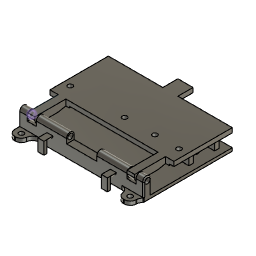
assembly (Autodesk Fusion 360 archive; units mm, degrees)
design "bottom"
Autodesk Fusion 360 part; units mm, degrees
(part 1 of 2)
sketch "Sketch1" plane through (0, 0, 0) normal (0, 0, 1) x (1, 0, 0)
  line L0 (325.5222, -11.5288) -> (325.5222, -23.0288)
  line L1 (309.5222, -20.1288) -> (309.5222, -14.4288)
  line L2 (192.5197, -2.0788) -> (192.5197, -69.9533) construction
  line L3 (325.5222, -11.5288) -> (316.5222, -11.5288)
  line L4 (325.5222, -23.0288) -> (316.5222, -23.0288)
  line L5 (334.5222, -14.4288) -> (343.2222, -14.4288)
  line L6 (350.5222, -11.5288) -> (350.5222, -23.0288)
  line L7 (334.5222, -20.1288) -> (334.5222, -14.4288)
  line L8 (343.2222, -20.1288) -> (343.2222, -23.0288)
  line L9 (350.5222, -11.5288) -> (343.2222, -11.5288)
  line L10 (343.2222, -14.4288) -> (343.2222, -11.5288)
  line L11 (334.5222, -20.1288) -> (343.2222, -20.1288)
  line L12 (350.5222, -23.0288) -> (343.2222, -23.0288)
  line L13 (367.5222, -87.072) -> (367.5222, -157.1728)
  line L14 (327.5222, -47.072) -> (317.8871, -47.072)
  line L15 (312.8871, -42.072) -> (312.8871, -37.072)
  line L16 (317.8871, -32.072) -> (372.5422, -32.072)
  arc A0 (317.8871, -32.072) -> (312.8871, -37.072) centre (317.8871, -37.072) ccw
  arc A1 (312.8871, -42.072) -> (317.8871, -47.072) centre (317.8871, -42.072) ccw
  arc A2 (367.5222, -87.072) -> (327.5222, -47.072) centre (327.5222, -87.072) ccw
  arc A3 (284.5222, -240.1728) -> (367.5222, -157.1728) centre (284.5222, -157.1728) ccw
  line L17 (67.1522, -32.072) -> (12.4972, -32.072)
  arc A4 (72.1522, -37.072) -> (67.1522, -32.072) centre (67.1522, -37.072) ccw
  line L18 (72.1522, -42.072) -> (72.1522, -37.072)
  arc A5 (67.1522, -47.072) -> (72.1522, -42.072) centre (67.1522, -42.072) ccw
  line L19 (57.5171, -47.072) -> (67.1522, -47.072)
  arc A6 (57.5171, -47.072) -> (17.5171, -87.072) centre (57.5171, -87.072) ccw
  line L20 (17.5171, -87.072) -> (17.5171, -157.1728)
  arc A7 (17.5171, -157.1728) -> (100.5171, -240.1728) centre (100.5171, -157.1728) ccw
  line L21 (316.5222, -11.5288) -> (314.4916, -14.4288)
  line L22 (316.5222, -11.5288) -> (320.409, -11.5288) construction
  line L23 (309.5222, -20.1288) -> (314.4916, -20.1288)
  line L24 (314.4916, -20.1288) -> (316.5222, -23.0288)
  line L25 (314.4916, -14.4288) -> (309.5222, -14.4288)
  circle A8 centre (362.5222, -10.5788) radius 3
  circle A9 centre (362.5222, -23.572) radius 3
  circle A10 centre (373.5222, -17.0788) radius 4
  line L26 (360.5472, -12.837) -> (360.5472, -21.3138)
  circle A11 centre (278.8372, -196.4356) radius 3
  circle A12 centre (278.8372, -209.4287) radius 3
  circle A13 centre (267.8372, -202.9356) radius 4
  line L27 (280.8122, -198.6937) -> (280.8122, -207.1706)
  circle A14 centre (253.8372, -209.4287) radius 3
  circle A15 centre (253.8372, -196.4356) radius 3
  circle A16 centre (242.8372, -202.9356) radius 4
  line L28 (255.8122, -198.6937) -> (255.8122, -207.1706)
  circle A17 centre (303.8372, -209.4287) radius 3
  circle A18 centre (303.8372, -196.4356) radius 3
  circle A19 centre (292.8372, -202.9356) radius 4
  line L29 (305.8122, -198.6937) -> (305.8122, -207.1706)
  line L30 (372.5422, -32.072) -> (372.5222, -32.072)
  line L31 (382.5222, -22.072) -> (382.5222, -12.0576)
  line L32 (372.5222, -2.0576) -> (372.5422, -2.0576)
  arc A20 (382.5222, -12.0576) -> (372.5222, -2.0576) centre (372.5222, -12.0576) ccw
  arc A21 (372.5222, -32.072) -> (382.5222, -22.072) centre (372.5222, -22.072) ccw
  arc A22 (12.5171, -2.0576) -> (2.5171, -12.0576) centre (12.5171, -12.0576) ccw
  line L33 (2.5171, -22.072) -> (2.5171, -12.0576)
  arc A23 (2.5171, -22.072) -> (12.5171, -32.072) centre (12.5171, -22.072) ccw
  line L34 (284.5222, -240.1728) -> (100.5171, -240.1728)
  line L35 (12.5171, -2.0576) -> (372.5422, -2.0576)
  line L36 (133.9354, -11.0576) -> (139.9354, -11.0576)
  line L37 (142.3054, -15.8969) -> (141.8063, -16.54)
  line L38 (144.1763, -21.3793) -> (157.1763, -21.3793)
  line L39 (159.6876, -16.7381) -> (159.0084, -15.6988)
  line L40 (161.5197, -11.0576) -> (167.5197, -11.0576)
  arc A24 (142.3054, -15.8969) -> (139.9354, -11.0576) centre (139.9354, -14.0576) ccw
  arc A25 (161.5197, -11.0576) -> (159.0084, -15.6988) centre (161.5197, -14.0576) ccw
  arc A26 (157.1763, -21.3793) -> (159.6876, -16.7381) centre (157.1763, -18.3793) ccw
  arc A27 (141.8063, -16.54) -> (144.1763, -21.3793) centre (144.1763, -18.3793) ccw
  arc A28 (226.0309, -15.6988) -> (223.5197, -11.0576) centre (223.5197, -14.0576) ccw
  arc A29 (240.863, -21.3793) -> (243.233, -16.54) centre (240.863, -18.3793) ccw
  line L41 (240.863, -21.3793) -> (227.863, -21.3793)
  line L42 (242.7339, -15.8969) -> (243.233, -16.54)
  arc A30 (245.1039, -11.0576) -> (242.7339, -15.8969) centre (245.1039, -14.0576) ccw
  line L43 (223.5197, -11.0576) -> (217.5197, -11.0576)
  line L44 (225.3517, -16.7381) -> (226.0309, -15.6988)
  line L45 (251.1039, -11.0576) -> (245.1039, -11.0576)
  arc A31 (225.3517, -16.7381) -> (227.863, -21.3793) centre (227.863, -18.3793) ccw
  line L46 (315.4335, -32.7154) -> (320, -31)
  line L47 (242.8372, -198.9356) -> (242.8372, -206.9356) construction
  line L48 (238.8372, -202.9356) -> (246.8372, -202.9356) construction
  line L49 (250.8372, -196.4356) -> (256.8372, -196.4356) construction
  line L50 (253.8372, -193.4356) -> (253.8372, -199.4356) construction
  line L51 (253.8372, -206.4287) -> (253.8372, -212.4287) construction
  line L52 (250.8372, -209.4287) -> (256.8372, -209.4287) construction
  line L53 (263.8372, -202.9356) -> (271.8372, -202.9356) construction
  line L54 (267.8372, -198.9356) -> (267.8372, -206.9356) construction
  line L55 (275.8372, -196.4356) -> (281.8372, -196.4356) construction
  line L56 (278.8372, -193.4356) -> (278.8372, -199.4356) construction
  line L57 (278.8372, -206.4287) -> (278.8372, -212.4287) construction
  line L58 (275.8372, -209.4287) -> (281.8372, -209.4287) construction
  line L59 (288.8372, -202.9356) -> (296.8372, -202.9356) construction
  line L60 (292.8372, -198.9356) -> (292.8372, -206.9356) construction
  line L61 (300.8372, -196.4356) -> (306.8372, -196.4356) construction
  line L62 (303.8372, -193.4356) -> (303.8372, -199.4356) construction
  line L63 (303.8372, -206.4287) -> (303.8372, -212.4287) construction
  line L64 (300.8372, -209.4287) -> (306.8372, -209.4287) construction
  line L65 (92.2021, -198.9356) -> (92.2021, -206.9356) construction
  line L66 (109.2021, -209.4287) -> (103.2021, -209.4287) construction
  line L67 (142.2021, -198.9356) -> (142.2021, -206.9356) construction
  line L68 (131.2021, -206.4287) -> (131.2021, -212.4287) construction
  line L69 (109.2021, -196.4356) -> (103.2021, -196.4356) construction
  line L70 (131.2021, -193.4356) -> (131.2021, -199.4356) construction
  circle A32 centre (131.2021, -196.4356) radius 3
  circle A33 centre (142.2021, -202.9356) radius 4
  circle A34 centre (117.2021, -202.9356) radius 4
  line L71 (104.2271, -198.6937) -> (104.2271, -207.1706)
  line L72 (81.2021, -193.4356) -> (81.2021, -199.4356) construction
  line L73 (106.2021, -206.4287) -> (106.2021, -212.4287) construction
  line L74 (106.2021, -193.4356) -> (106.2021, -199.4356) construction
  line L75 (96.2021, -202.9356) -> (88.2021, -202.9356) construction
  line L76 (134.2021, -196.4356) -> (128.2021, -196.4356) construction
  line L77 (79.2271, -198.6937) -> (79.2271, -207.1706)
  line L78 (117.2021, -198.9356) -> (117.2021, -206.9356) construction
  circle A35 centre (106.2021, -196.4356) radius 3
  line L79 (81.2021, -206.4287) -> (81.2021, -212.4287) construction
  line L80 (134.2021, -209.4287) -> (128.2021, -209.4287) construction
  circle A36 centre (81.2021, -196.4356) radius 3
  circle A37 centre (92.2021, -202.9356) radius 4
  line L81 (84.2021, -209.4287) -> (78.2021, -209.4287) construction
  circle A38 centre (131.2021, -209.4287) radius 3
  line L82 (84.2021, -196.4356) -> (78.2021, -196.4356) construction
  line L83 (129.2271, -198.6937) -> (129.2271, -207.1706)
  circle A39 centre (106.2021, -209.4287) radius 3
  line L84 (146.2021, -202.9356) -> (138.2021, -202.9356) construction
  circle A40 centre (81.2021, -209.4287) radius 3
  line L85 (121.2021, -202.9356) -> (113.2021, -202.9356) construction
  line L86 (362.5222, -20.572) -> (362.5222, -26.572) construction
  line L87 (359.5222, -23.572) -> (365.5222, -23.572) construction
  line L88 (373.5221, -13.0788) -> (373.5221, -21.0788) construction
  line L89 (369.5222, -17.0788) -> (377.5222, -17.0788) construction
  line L90 (362.5222, -7.5788) -> (362.5222, -13.5788) construction
  line L91 (359.5222, -10.5788) -> (365.5222, -10.5788) construction
  line L92 (59.5171, -23.0288) -> (68.5171, -23.0288)
  line L93 (22.5171, -20.572) -> (22.5171, -26.572) construction
  line L94 (11.5172, -13.0788) -> (11.5172, -21.0788) construction
  line L95 (34.5171, -11.5288) -> (41.8171, -11.5288)
  line L96 (25.5171, -10.5788) -> (19.5171, -10.5788) construction
  line L97 (34.5171, -23.0288) -> (41.8171, -23.0288)
  line L98 (59.5171, -11.5288) -> (68.5171, -11.5288)
  line L99 (34.5171, -11.5288) -> (34.5171, -23.0288)
  circle A41 centre (22.5171, -23.572) radius 3
  circle A42 centre (11.5171, -17.0788) radius 4
  line L100 (75.5171, -20.1288) -> (75.5171, -14.4288)
  line L101 (25.5171, -23.572) -> (19.5171, -23.572) construction
  line L102 (50.5171, -14.4288) -> (41.8171, -14.4288)
  line L103 (68.5171, -11.5288) -> (64.6303, -11.5288) construction
  line L104 (70.5477, -14.4288) -> (75.5171, -14.4288)
  line L105 (70.5477, -20.1288) -> (68.5171, -23.0288)
  line L106 (22.5171, -7.5788) -> (22.5171, -13.5788) construction
  line L107 (75.5171, -20.1288) -> (70.5477, -20.1288)
  line L108 (41.8171, -20.1288) -> (41.8171, -23.0288)
  line L109 (68.5171, -11.5288) -> (70.5477, -14.4288)
  line L110 (24.4921, -12.837) -> (24.4921, -21.3138)
  line L111 (15.5171, -17.0788) -> (7.5171, -17.0788) construction
  line L112 (50.5171, -20.1288) -> (41.8171, -20.1288)
  line L113 (50.5171, -20.1288) -> (50.5171, -14.4288)
  line L114 (59.5171, -11.5288) -> (59.5171, -23.0288)
  circle A43 centre (22.5171, -10.5788) radius 3
  line L115 (41.8171, -14.4288) -> (41.8171, -11.5288)
  point P0 (309.5222, -17.2788)
  point P1 (325.5222, -17.2788)
  point P2 (325.5222, -17.2788)
  point P3 (309.5222, -17.2788)
  point P4 (350.5222, -17.2788)
  point P5 (334.5222, -17.2788)
  point P6 (350.5222, -17.2788)
  point P7 (334.5222, -17.2788)
  point P8 (330.5222, -17.0788)
  point P9 (314.5222, -17.0788)
  point P10 (330.5222, -17.0788)
  point P11 (314.5222, -17.0788)
  point P12 (359.5472, -10.1923)
  point P13 (359.5433, -23.9267)
  point P14 (281.8162, -209.7835)
  point P15 (281.8122, -196.0491)
  point P16 (256.8122, -196.0491)
  point P17 (256.8162, -209.7835)
  point P18 (306.8122, -196.0491)
  point P19 (306.8162, -209.7835)
  point P20 (192.5197, -240.1728)
  point P21 (128.2231, -209.7835)
  point P22 (78.2271, -196.0491)
  point P23 (103.2271, -196.0491)
  point P24 (103.2231, -209.7835)
  point P25 (128.2271, -196.0491)
  point P26 (78.2231, -209.7835)
  point P27 (59.5171, -17.2788)
  point P28 (54.5171, -17.0788)
  point P29 (12.5171, -22.072)
  point P30 (59.5171, -17.2788)
  point P31 (34.5171, -17.2788)
  point P32 (50.5171, -17.2788)
  point P33 (70.5171, -17.0788)
  point P34 (70.5171, -17.0788)
  point P35 (34.5171, -17.2788)
  point P36 (50.5171, -17.2788)
  point P37 (12.5171, -12.0576)
  point P38 (25.4921, -10.1923)
  point P39 (25.496, -23.9267)
  point P40 (75.5171, -17.2788)
  point P41 (75.5171, -17.2788)
  point P42 (54.5171, -17.0788)
  dimension "d16" = 5.7
  dimension "d20" = 11.5
  dimension "d25" = 16
  dimension "d27" = 9
  dimension "d28" = 9
  dimension "d33" = 5.7
  dimension "d34" = 11.5
  dimension "d35" = 16
  dimension "d36" = 7.3
  dimension "d37" = 7.3
  dimension "d39" = 25
  dimension "d48" = 5
  dimension "d49" = 5
  dimension "d50" = 40
  dimension "d57" = 15
  dimension "d67" = 125
  dimension "d68" = 125
  dimension "d80" = 6
  dimension "d81" = 6
  dimension "d83" = 8.5
  dimension "d85" = 8
  dimension "d95" = 1
  dimension "d98" = 25
  dimension "d99" = 0
  dimension "d101" = 10
  dimension "d102" = 10
  dimension "d122" = 32
  dimension "d123" = 3
  dimension "d124" = 3
  dimension "d125" = 3
  dimension "d126" = 3
  dimension "d127" = 9
  dimension "d128" = 9
  dimension "d129" = 6
  dimension "d130" = 6
  dimension "d131" = 13
  constraint vertical L0
  constraint vertical L1
  constraint midpoint L1 P3
  constraint midpoint L0 P2
  constraint coincident P2 P1
  constraint coincident P3 P0
  constraint horizontal P2 P3
  constraint perpendicular L0 L3
  constraint perpendicular L0 L4
  constraint vertical L6
  constraint vertical L7
  constraint midpoint P7 L7
  constraint midpoint P6 L6
  constraint coincident P6 P4
  constraint coincident P7 P5
  constraint horizontal P6 P7
  constraint perpendicular L6 L9
  constraint perpendicular L6 L12
  constraint perpendicular L7 L11
  constraint perpendicular L8 L12
  constraint perpendicular L5 L7
  constraint perpendicular L9 L10
  constraint coincident P10 P8
  constraint coincident P11 P9
  constraint horizontal P10 P11
  constraint perpendicular L15 L16
  constraint perpendicular L14 L15
  constraint tangent L15 A0
  constraint tangent L16 A0
  constraint tangent L15 A1
  constraint tangent L14 A1
  constraint tangent L13 A2
  constraint tangent L14 A2
  constraint horizontal L16
  constraint tangent L13 A3
  constraint symmetric L16.end L2 L17.end
  constraint symmetric L2 L15.end A4.start
  constraint symmetric L2 L16.start L17.start
  constraint symmetric L2 A0 A4
  constraint symmetric L2 L15.start L18.start
  constraint symmetric L2 L14.end A5.start
  constraint symmetric L2 A1 A5
  constraint symmetric L2 L13.start A6.end
  constraint symmetric L2 L14.start L19.start
  constraint symmetric L2 A2 A6
  constraint symmetric L2 L13.end L20.end
  constraint symmetric L2 A3.start A7.end
  constraint symmetric L2 A3 A7
  constraint horizontal L22
  constraint perpendicular L1 L23
  constraint perpendicular L1 L25
  constraint vertical A8.centre A9.centre
  constraint coincident A8 P12
  constraint coincident A9 P13
  constraint coincident A8 L26.start
  constraint coincident A9 L26.end
  constraint vertical L26
  constraint perpendicular L31 L32
  constraint tangent L31 A20
  constraint tangent L32 A20
  constraint tangent L30 A21
  constraint tangent L31 A21
  constraint symmetric L2 L31.end A22.end
  constraint symmetric L2 L32.start A22.start
  constraint symmetric L2 A20 A22
  constraint symmetric L2 L30.end A23.end
  constraint symmetric L2 L31.start L33.start
  constraint symmetric L2 A21 A23
  constraint tangent A7 L34
  constraint tangent A20 L35
  constraint midpoint L34 P20
  constraint horizontal L36
  constraint parallel L36 L38
  constraint parallel L38 L40
  constraint tangent L36 A24
  constraint tangent L37 A24
  constraint tangent L40 A25
  constraint tangent L39 A25
  constraint tangent L38 A26
  constraint tangent L39 A26
  constraint tangent L37 A27
  constraint tangent L38 A27
  constraint symmetric L2 L36.start L45.start
  constraint symmetric L2 L40.end L43.end
  constraint symmetric L2 L36.end A30.start
  constraint symmetric L2 L37.start L42.start
  constraint symmetric L2 A24 A30
  constraint symmetric L2 L40.start A28.end
  constraint symmetric L2 L39.end A28.start
  constraint symmetric L2 A25 A28
  constraint symmetric L2 L38.end L41.end
  constraint symmetric L2 L39.start L44.start
  constraint symmetric L2 A26 A31
  constraint symmetric L2 L37.end A29.end
  constraint symmetric L2 L38.start A29.start
  constraint symmetric L2 A27 A29
  constraint coincident A0 L46.start
  constraint coincident A16 L47.start
  constraint coincident A16 L47.end
  constraint vertical L47
  constraint coincident A16 L48.start
  constraint coincident A16 L48.end
  constraint perpendicular L47 L48
  constraint coincident A15 L49.start
  constraint coincident A15 L49.end
  constraint horizontal L49
  constraint coincident A15 L50.start
  constraint coincident A15 L50.end
  constraint perpendicular L49 L50
  constraint coincident A14 L51.start
  constraint coincident A14 L51.end
  constraint parallel L28 L51
  constraint coincident A14 L52.start
  constraint coincident A14 L52.end
  constraint perpendicular L51 L52
  constraint coincident A13 L53.start
  constraint coincident A13 L53.end
  constraint horizontal L53
  constraint coincident A13 L54.start
  constraint coincident A13 L54.end
  constraint perpendicular L53 L54
  constraint coincident A11 L55.start
  constraint coincident A11 L55.end
  constraint horizontal L55
  constraint coincident A11 L56.start
  constraint coincident A11 L56.end
  constraint perpendicular L55 L56
  constraint coincident A12 L57.start
  constraint coincident A12 L57.end
  constraint perpendicular L55 L57
  constraint coincident A12 L58.start
  constraint coincident A12 L58.end
  constraint perpendicular L57 L58
  constraint coincident A19 L59.start
  constraint coincident A19 L59.end
  constraint horizontal L59
  constraint coincident A19 L60.start
  constraint coincident A19 L60.end
  constraint perpendicular L59 L60
  constraint coincident A18 L61.start
  constraint coincident A18 L61.end
  constraint horizontal L61
  constraint coincident A18 L62.start
  constraint coincident A18 L62.end
  constraint perpendicular L61 L62
  constraint coincident A17 L63.start
  constraint coincident A17 L63.end
  constraint perpendicular L61 L63
  constraint coincident A17 L64.start
  constraint coincident A17 L64.end
  constraint perpendicular L63 L64
  constraint symmetric L2 L27.start L71.start
  constraint symmetric L2 L27.end L71.end
  constraint symmetric L2 P14 P24
  constraint symmetric L2 P15 P23
  constraint symmetric L2 A11 A35
  constraint symmetric L2 A12 A39
  constraint symmetric L2 A13 A34
  constraint symmetric L2 L28.end L83.end
  constraint symmetric L2 P16 P25
  constraint symmetric L2 A14 A38
  constraint symmetric L2 L28.start L83.start
  constraint symmetric L2 A15 A32
  constraint symmetric L2 A16 A33
  constraint symmetric L2 P17 P21
  constraint symmetric L2 L29.end L77.end
  constraint symmetric L2 P18 P22
  constraint symmetric L2 A17 A40
  constraint symmetric L2 L29.start L77.start
  constraint symmetric L2 A18 A36
  constraint symmetric L2 A19 A37
  constraint symmetric L2 P19 P26
  constraint symmetric L2 L47.start L67.start
  constraint symmetric L2 L47.end L67.end
  constraint symmetric L2 L48.start L84.start
  constraint symmetric L2 L48.end L84.end
  constraint symmetric L2 L49.start L76.start
  constraint symmetric L2 L49.end L76.end
  constraint symmetric L2 L50.start L70.start
  constraint symmetric L2 L50.end L70.end
  constraint symmetric L2 L51.start L68.start
  constraint symmetric L2 L51.end L68.end
  constraint symmetric L2 L52.start L80.start
  constraint symmetric L2 L52.end L80.end
  constraint symmetric L2 L53.start L85.start
  constraint symmetric L2 L53.end L85.end
  constraint symmetric L2 L54.start L78.start
  constraint symmetric L2 L54.end L78.end
  constraint symmetric L2 L55.start L69.start
  constraint symmetric L2 L55.end L69.end
  constraint symmetric L2 L56.start L74.start
  constraint symmetric L2 L56.end L74.end
  constraint symmetric L2 L57.start L73.start
  constraint symmetric L2 L57.end L73.end
  constraint symmetric L2 L58.start L66.start
  constraint symmetric L2 L58.end L66.end
  constraint symmetric L2 L59.start L75.start
  constraint symmetric L2 L59.end L75.end
  constraint symmetric L2 L60.start L65.start
  constraint symmetric L2 L60.end L65.end
  constraint symmetric L2 L61.start L82.start
  constraint symmetric L2 L61.end L82.end
  constraint symmetric L2 L62.start L72.start
  constraint symmetric L2 L62.end L72.end
  constraint symmetric L2 L63.start L79.start
  constraint symmetric L2 L63.end L79.end
  constraint symmetric L2 L64.start L81.start
  constraint symmetric L2 L64.end L81.end
  constraint coincident A9 L86.start
  constraint coincident A9 L86.end
  constraint vertical L86
  constraint coincident A9 L87.start
  constraint coincident A9 L87.end
  constraint perpendicular L86 L87
  constraint coincident A10 L88.start
  constraint coincident A10 L88.end
  constraint perpendicular L87 L88
  constraint coincident A10 L89.start
  constraint coincident A10 L89.end
  constraint perpendicular L88 L89
  constraint coincident A8 L90.start
  constraint coincident A8 L90.end
  constraint vertical L90
  constraint coincident A8 L91.start
  constraint coincident A8 L91.end
  constraint perpendicular L90 L91
  constraint symmetric L1.end L2 L100.end
  constraint symmetric L0.start L2 L98.start
  constraint symmetric L1.start L2 L100.start
  constraint symmetric L2 L0.end L92.start
  constraint symmetric L2 P3 P41
  constraint symmetric L2 P2 P30
  constraint symmetric L2 L3.end L98.end
  constraint symmetric L2 L4.end L92.end
  constraint symmetric L2 P6 P35
  constraint symmetric L2 L6.start L95.start
  constraint symmetric L2 L5.start L102.start
  constraint symmetric L2 L7.start L112.start
  constraint symmetric L2 L6.end L97.start
  constraint symmetric L2 P7 P36
  constraint symmetric L2 L5.end L102.end
  constraint symmetric L2 L8.start L108.start
  constraint symmetric L2 L8.end L97.end
  constraint symmetric L2 L9.end L95.end
  constraint symmetric L2 P10 P42
  constraint symmetric L2 P11 P34
  constraint symmetric L2 L21.end L104.start
  constraint symmetric L2 L22.end L103.end
  constraint symmetric L2 L23.end L105.start
  constraint symmetric L2 A8 A43
  constraint symmetric L2 A9 A41
  constraint symmetric L2 A10 A42
  constraint symmetric L2 P12 P38
  constraint symmetric L2 P13 P39
  constraint symmetric L2 L26.start L110.start
  constraint symmetric L2 L26.end L110.end
  constraint symmetric L2 A20.centre P37
  constraint symmetric L2 A21.centre P29
  constraint symmetric L2 L86.start L93.start
  constraint symmetric L2 L86.end L93.end
  constraint symmetric L2 L87.start L101.start
  constraint symmetric L2 L87.end L101.end
  constraint symmetric L2 L88.start L94.start
  constraint symmetric L2 L88.end L94.end
  constraint symmetric L2 L89.start L111.start
  constraint symmetric L2 L89.end L111.end
  constraint symmetric L2 L90.start L106.start
  constraint symmetric L2 L90.end L106.end
  constraint symmetric L2 L91.start L96.start
  constraint symmetric L2 L91.end L96.end
  measures "d16" distance of L1.end L1.start
  measures "d20" distance of L0.start L0.end
  measures "d25" distance of L0 L1
  measures "d27" distance of L0.start L3.end
  measures "d28" distance of L0.end L4.end
  measures "d33" distance of L5.start L7.start
  measures "d34" distance of L6.start L6.end
  measures "d35" distance of L6 L7
  measures "d36" distance of L6.start L9.end
  measures "d37" distance of L6.end L8.end
  measures "d39" distance of L0.end L6.end
  measures "d48" radius of A0
  measures "d49" radius of A1
  measures "d50" radius of A2
  measures "d57" distance of L14 L16
  measures "d67" angle of L21 L22
  measures "d68" angle of L4 L24
  measures "d80" diameter of A8
  measures "d81" diameter of A9
  measures "d83" distance of L16 A9.centre
  measures "d85" diameter of A10
  measures "d95" distance of P12 L26
  measures "d101" radius of A20
  measures "d102" radius of A21
  measures "d122" distance of L6 L31
  measures "d123" radius of A24
  measures "d124" radius of A25
  measures "d125" radius of A26
  measures "d126" radius of A27
  measures "d127" distance of L35 L36
  measures "d128" distance of L35 L40
  measures "d129" distance of L36.start L36.end
  measures "d130" distance of L40.end L40.start
  measures "d131" distance of L38.end L38.start
sketch "Sketch2" plane through (0, 0, 0) normal (0, 0, 1) x (1, 0, 0)
  circle A0 centre (81.2021, -196.4356) radius 3
  circle A1 centre (81.2021, -209.4287) radius 3
  circle A2 centre (92.2021, -202.9356) radius 4
  circle A3 centre (106.2021, -196.4356) radius 3
  circle A4 centre (106.2021, -209.4287) radius 3
  circle A5 centre (117.2021, -202.9356) radius 4
  circle A6 centre (131.2021, -196.4356) radius 3
  circle A7 centre (131.2021, -209.4287) radius 3
  circle A8 centre (142.2021, -202.9356) radius 4
  line L0 (79.2271, -198.6937) -> (79.2271, -207.1706)
  line L1 (104.2271, -198.6937) -> (104.2271, -207.1706)
  line L2 (129.2271, -198.6937) -> (129.2271, -207.1706)
  circle A9 centre (81.2021, -196.4356) radius 2.8
  circle A10 centre (81.2021, -209.4287) radius 2.8
  circle A11 centre (92.2021, -202.9356) radius 3.8
  circle A12 centre (106.2021, -196.4356) radius 2.8
  circle A13 centre (106.2021, -209.4287) radius 2.8
  circle A14 centre (117.2021, -202.9356) radius 3.8
  circle A15 centre (131.2021, -209.4287) radius 2.8
  circle A16 centre (131.2021, -196.4356) radius 2.8
  circle A17 centre (142.2021, -202.9356) radius 3.8
  dimension "d152" = -0.2
  dimension "d154" = 0.2
  dimension "d155" = 0.2
  constraint concentric A1 A10
  constraint concentric A2 A11
  constraint concentric A3 A12
  constraint concentric A4 A13
  constraint concentric A5 A14
  constraint concentric A7 A15
  constraint concentric A6 A16
  constraint concentric A8 A17
  constraint equal A9 A10
  constraint equal A9 A12
  constraint equal A9 A13
  constraint equal A9 A16
  constraint equal A9 A15
  constraint equal A14 A17
  measures "d154" distance of A2 A11
  measures "d155" distance of A5 A14
extrude "Extrude1" add sketch "Sketch2" along normal blind 5 contours A9 | A10 | A11 | A12 | A13 | A14 | A15 | A16 | A17 makes body 1 at (132.3537, -193.8834, 1.6667) makes body 2 at (95.7729, -204.2352, 3.3333) makes body 3 at (79.5676, -211.7022, 3.3333) makes body 4 at (120.7729, -204.2352, 3.3333) makes body 5 at (132.3537, -206.8765, 1.6667) makes body 6 at (104.5676, -198.709, 3.3333) makes body 7 at (79.5676, -198.709, 3.3333) makes body 8 at (104.5676, -211.7022, 3.3333) makes body 9 at (144.7165, -200.0864, 3.3333)
sketch "Sketch3" plane through (0, 0, 0) normal (0, 0, 1) x (1, 0, 0)
  line L0 (72, -219) -> (154, -219)
  line L1 (154, -219) -> (154, -188)
  line L2 (154, -188) -> (72, -188)
  line L3 (72, -188) -> (72, -219)
  constraint horizontal L0
  constraint vertical L1
  constraint horizontal L2
  constraint vertical L3
extrude "Extrude2" add sketch "Sketch3" against normal blind 2 bodies 1 2 3 4 5 6 7 8 9
sketch "Sketch4" plane through (0, -219, 0) normal (0, -1, 0) x (1, 0, 0)
  line L0 (154, 0) -> (72, 0)
  line L1 (72, 0) -> (72, -2)
  line L2 (72, -2) -> (154, -2)
  line L3 (154, -2) -> (154, 0)
  line L4 (79.2271, 0) -> (79.7271, 0)
  line L5 (79.7271, 0) -> (79.7271, 3)
  line L6 (79.7271, 3) -> (80.7271, 3)
  arc A0 (80.7271, 3) -> (83.7271, 0) centre (83.7271, 3) ccw
  line L7 (72.0189, 0) -> (311.5187, 0)
  line L8 (80.7271, 3) -> (80.7271, 3.3) construction
  line L9 (83.7271, 0) -> (79.7271, 0)
  point P0 (129.2271, 0)
  point P1 (104.2271, 0)
  point P2 (79.2271, 0)
  dimension "d163" = 0.5
  dimension "d164" = 3
  dimension "d165" = 1
  constraint coincident P2 L4.start
  constraint parallel L0 L4
  constraint perpendicular L4 L5
  constraint perpendicular L5 L6
  constraint coincident L0 A0.end
  constraint tangent A0 L7
  constraint perpendicular L6 L8
  constraint tangent A0 L8
  measures "d163" distance of P2 L4.end
  measures "d164" distance of L4.end L5.end
  measures "d165" distance of L5.end L6.end
extrude "Extrude4" add sketch "Sketch4" against normal blind 6 from surface at -13 separate body contours L0 L5 L6 A0 L7 L9 makes body 10
copy_body "CopyPasteBodies2" bodies 10 makes body 11
move_body "Move1" bodies 11 to x (1, 0, 0) y (0, 1, 0) z (0, 0, 1) at (25, 0, 0)
copy_body "CopyPasteBodies3" bodies 10 makes body 12
move_body "Move2" bodies 12 to x (1, 0, 0) y (0, 1, 0) z (0, 0, 1) at (50, 0, 0)
combine "Combine1" operation add target body 1 tool bodies 10 11 12
extrude "Extrude10" add 2 faces at (90.7094, -201.9453, 5) (142.484, -204.1705, 5) along direction (0, 0, 1) blind 3 on bodies 1 bodies 1
chamfer "Chamfer1" distance 2 distance2 3 7 edges at (78.5916, -197.4481, 5) (78.5916, -210.4413, 5) (103.5916, -210.4413, 5) (103.5916, -197.4481, 5) (113.6593, -204.3097, 5) (128.5916, -210.4413, 5) (128.5916, -197.4481, 5) measured on face at (81.4098, -197.3455, 5) measured on face at (81.4098, -210.3387, 5) measured on face at (106.4098, -210.3387, 5) measured on face at (106.4098, -197.3455, 5) measured on face at (115.7094, -201.9453, 5) measured on face at (130.8611, -210.2976, 5) measured on face at (130.8611, -197.3044, 5) on bodies 1 3 4 5 6 7 8
chamfer "Chamfer2" distance 3 distance2 4 2 edges at (88.6593, -204.3097, 8) (138.6593, -204.3097, 8) measured on face at (90.7094, -201.9453, 8) measured on face at (142.484, -204.1705, 8) on bodies 1
sketch "Sketch10" plane through (0, 0, 0) normal (0, 0, 1) x (-1, 0, 0)
  line L0 (-133.7271, 200) -> (-133.7271, 206)
  line L1 (-133.7271, 206) -> (-129.7271, 206)
  line L2 (-129.7271, 206) -> (-129.7271, 200)
  line L3 (-129.7271, 200) -> (-133.7271, 200)
  line L4 (-108.7271, 200) -> (-108.7271, 206)
  line L5 (-108.7271, 206) -> (-104.7271, 206)
  line L6 (-104.7271, 206) -> (-104.7271, 200)
  line L7 (-104.7271, 200) -> (-108.7271, 200)
  line L8 (-83.7271, 200) -> (-83.7271, 206)
  line L9 (-83.7271, 206) -> (-79.7271, 206)
  line L10 (-79.7271, 206) -> (-79.7271, 200)
  line L11 (-79.7271, 200) -> (-83.7271, 200)
  circle A0 centre (-142.2021, 202.9356) radius 3.8
  circle A1 centre (-106.2021, 209.4287) radius 2.8
  circle A2 centre (-81.2021, 196.4356) radius 2.8
  circle A3 centre (-106.2021, 196.4356) radius 2.8
  circle A4 centre (-131.2021, 209.4287) radius 2.8
  circle A5 centre (-117.2021, 202.9356) radius 3.8
  circle A6 centre (-81.2021, 209.4287) radius 2.8
  circle A7 centre (-92.2021, 202.9356) radius 3.8
  line L12 (-72, 188) -> (-72, 219)
  line L13 (-72, 219) -> (-154, 219)
  line L14 (-154, 219) -> (-154, 188)
  line L15 (-154, 188) -> (-72, 188)
  circle A8 centre (-131.2021, 196.4356) radius 2.8
  arc A9 (-17.5171, 157.1728) -> (-100.5171, 240.1728) centre (-100.5171, 157.1728) ccw
  line L16 (-284.5222, 240.1728) -> (-100.5171, 240.1728)
  arc A10 (-16.0171, 157.1728) -> (-100.5171, 241.6728) centre (-100.5171, 157.1728) ccw
  line L17 (-284.5222, 241.6728) -> (-100.5171, 241.6728)
  line L18 (-72, 219) -> (-72, 236.7154)
  line L19 (-154, 219) -> (-154, 241.6728)
  dimension "d197" = -1.5
  constraint coincident L12.end L13.start
  constraint coincident A10 L18.end
  constraint perpendicular L13 L18
  constraint coincident L13.end L14.start
  constraint coincident L17 L19.end
  constraint perpendicular L17 L19
extrude "Extrude11" add sketch "Sketch10" against normal up to surface (2 mm away) contours L13 A9 L16 L18 L19 | A9 L16 A10 L17 L18 L19 bodies 1
sketch "Sketch11" plane through (0, 0, 0) normal (0, 0, 1) x (-1, 0, 0)
  line L0 (-133.7271, 200) -> (-133.7271, 206)
  line L1 (-133.7271, 206) -> (-129.7271, 206)
  line L2 (-129.7271, 206) -> (-129.7271, 200)
  line L3 (-129.7271, 200) -> (-133.7271, 200)
  line L4 (-108.7271, 200) -> (-108.7271, 206)
  line L5 (-108.7271, 206) -> (-104.7271, 206)
  line L6 (-104.7271, 206) -> (-104.7271, 200)
  line L7 (-104.7271, 200) -> (-108.7271, 200)
  line L8 (-83.7271, 200) -> (-83.7271, 206)
  line L9 (-83.7271, 206) -> (-79.7271, 206)
  line L10 (-79.7271, 206) -> (-79.7271, 200)
  line L11 (-79.7271, 200) -> (-83.7271, 200)
  circle A0 centre (-142.2021, 202.9356) radius 3.8
  circle A1 centre (-106.2021, 209.4287) radius 2.8
  circle A2 centre (-81.2021, 196.4356) radius 2.8
  circle A3 centre (-106.2021, 196.4356) radius 2.8
  circle A4 centre (-131.2021, 209.4287) radius 2.8
  circle A5 centre (-117.2021, 202.9356) radius 3.8
  circle A6 centre (-81.2021, 209.4287) radius 2.8
  circle A7 centre (-92.2021, 202.9356) radius 3.8
  line L12 (-72, 188) -> (-72, 236.7154)
  arc A8 (-72, 236.7154) -> (-100.5171, 241.6728) centre (-100.5171, 157.1728) ccw
  line L13 (-100.5171, 241.6728) -> (-154, 241.6728)
  line L14 (-154, 241.6728) -> (-154, 188)
  line L15 (-154, 188) -> (-72, 188)
  circle A9 centre (-131.2021, 196.4356) radius 2.8
  line L16 (-100.5171, 241.6728) -> (-72, 241.6728)
  line L17 (-72, 241.6728) -> (-72, 236.7154)
  line L18 (-72, 241.6728) -> (-154, 241.6728)
  line L19 (-154, 241.6728) -> (-154, 246.6728)
  line L20 (-154, 246.6728) -> (-72, 246.6728)
  line L21 (-72, 246.6728) -> (-72, 241.6728)
  dimension "d200" = 5
  constraint coincident A8.end L13.start
  constraint tangent A8 L16
  constraint coincident L12.end A8.start
  constraint perpendicular L16 L17
  constraint horizontal L18
  constraint vertical L19
  constraint horizontal L20
  constraint vertical L21
  measures "d200" distance of L16.end L20.end
extrude "Extrude12" add sketch "Sketch11" along normal blind 6 and the other way up to surface (2 mm away) contours A8 L16 L17 L18 | L13 L16 L18 L19 L20 L21 bodies 1
sketch "Sketch12" plane through (154, 0, 0) normal (1, 0, 0) x (0, 1, 0)
  line L0 (-188, 0) -> (-241.6728, 0)
  line L1 (-241.6728, 0) -> (-241.6728, 6)
  line L2 (-241.6728, 6) -> (-246.6728, 6)
  line L3 (-246.6728, 6) -> (-246.6728, -2)
  line L4 (-246.6728, -2) -> (-188, -2)
  line L5 (-188, -2) -> (-188, 0)
  circle A0 centre (-244.1728, 9) radius 1.7
  line L6 (-246.6728, 6) -> (-244.1728, 9) construction
  line L7 (-244.1728, 9) -> (-241.6728, 6) construction
  line L8 (-246.6728, 6) -> (-246.6728, 9.1)
  arc A1 (-241.6728, 9.1) -> (-246.6728, 9.1) centre (-244.1728, 9.1) ccw
  line L9 (-241.6728, 9.1) -> (-241.6728, 6)
  dimension "d205" = 3.4
  dimension "d206" = 3
  dimension "d207" = 0.1
  constraint coincident L2.end L3.start
  constraint coincident A0.centre L6.end
  constraint coincident L1.end L2.start
  constraint equal L6 L7
  constraint perpendicular L2 L8
  constraint tangent L8 A1
  constraint tangent A1 L9
  constraint vertical L9
  measures "d205" diameter of A0
  measures "d206" distance of L2 A0.centre
  measures "d207" vertical distance of A0.centre A1.centre
extrude "Extrude13" add sketch "Sketch12" against normal blind 5 contours L2 L8 A1 L9 bodies 1
extrude "Extrude14" add 1 faces at (149, -244.2151, 6.4349) along direction (-1, 0, 0) blind 5 from surface at 6 on bodies 1 bodies 1
extrude "Extrude15" add 1 faces at (138, -244.2151, 6.4349) along direction (-1, 0, 0) blind 5 from surface at 61 on bodies 1 bodies 1
extrude "Extrude16" add 1 faces at (77, -244.2151, 6.4349) along direction (1, 0, 0) blind 5 from surface at 6 on bodies 1 bodies 1
sketch "Sketch1 (2)" plane through (0, 0, 6) normal (0, 0, 1) x (-1, 0, 0) in component "Component"
  line L0 (-83, 246.6728) -> (-83, 241.6728)
  line L1 (-83, 241.6728) -> (-88, 241.6728)
  line L2 (-88, 241.6728) -> (-88, 246.6728)
  line L3 (-88, 246.6728) -> (-138, 246.6728)
  line L4 (-138, 246.6728) -> (-138, 241.6728)
  line L5 (-138, 241.6728) -> (-100.5171, 241.6728)
  arc A0 (-72, 236.7154) -> (-100.5171, 241.6728) centre (-100.5171, 157.1728) ccw
  line L6 (-72, 236.7154) -> (-72, 241.6728)
  line L7 (-72, 241.6728) -> (-77, 241.6728)
  line L8 (-77, 241.6728) -> (-77, 246.6728)
  line L9 (-77, 246.6728) -> (-83, 246.6728)
  line L10 (-72, 226.6728) -> (-154, 226.6728)
  line L11 (-154, 226.6728) -> (-154, 188)
  line L12 (-154, 188) -> (-72, 188)
  line L13 (-72, 188) -> (-72, 226.6728)
  line L14 (-133.7271, 200) -> (-133.7271, 206)
  line L15 (-133.7271, 206) -> (-129.7271, 206)
  line L16 (-129.7271, 206) -> (-129.7271, 200)
  line L17 (-129.7271, 200) -> (-133.7271, 200)
  line L18 (-108.7271, 200) -> (-108.7271, 206)
  line L19 (-108.7271, 206) -> (-104.7271, 206)
  line L20 (-104.7271, 206) -> (-104.7271, 200)
  line L21 (-104.7271, 200) -> (-108.7271, 200)
  line L22 (-83.7271, 200) -> (-83.7271, 206)
  line L23 (-83.7271, 206) -> (-79.7271, 206)
  line L24 (-79.7271, 206) -> (-79.7271, 200)
  line L25 (-79.7271, 200) -> (-83.7271, 200)
  circle A1 centre (-142.2021, 202.9356) radius 3.8
  circle A2 centre (-106.2021, 209.4287) radius 2.8
  circle A3 centre (-81.2021, 196.4356) radius 2.8
  circle A4 centre (-106.2021, 196.4356) radius 2.8
  circle A5 centre (-131.2021, 209.4287) radius 2.8
  circle A6 centre (-117.2021, 202.9356) radius 3.8
  circle A7 centre (-81.2021, 209.4287) radius 2.8
  circle A8 centre (-92.2021, 202.9356) radius 3.8
  line L26 (-72, 188) -> (-72, 236.7154)
  arc A9 (-72, 236.7154) -> (-100.5171, 241.6728) centre (-100.5171, 157.1728) ccw
  line L27 (-100.5171, 241.6728) -> (-154, 241.6728)
  line L28 (-154, 241.6728) -> (-154, 188)
  line L29 (-154, 188) -> (-72, 188)
  circle A10 centre (-131.2021, 196.4356) radius 2.8
  line L30 (-143, 241.6728) -> (-143, 246.6728)
  line L31 (-143, 246.6728) -> (-149, 246.6728)
  line L32 (-149, 246.6728) -> (-149, 241.6728)
  line L33 (-149, 241.6728) -> (-143, 241.6728)
  line L34 (-77.5, 246.6728) -> (-82.5, 246.6728)
  line L35 (-82.5, 246.6728) -> (-82.5, 226.6728)
  line L36 (-82.5, 226.6728) -> (-77.5, 226.6728)
  line L37 (-77.5, 226.6728) -> (-77.5, 246.6728)
  line L38 (-143.5, 246.6728) -> (-148.5, 246.6728)
  line L39 (-148.5, 246.6728) -> (-148.5, 226.6728)
  line L40 (-148.5, 226.6728) -> (-143.5, 226.6728)
  line L41 (-143.5, 226.6728) -> (-143.5, 246.6728)
  point P0 (-72, 188)
  point P1 (-154, 188)
  dimension "d219" = 0.5
  dimension "d220" = 0.5
  dimension "d221" = 0.5
  dimension "d222" = 0.5
  dimension "d223" = 20
  constraint horizontal L10
  constraint vertical L11
  constraint horizontal L12
  constraint vertical L13
  constraint coincident P0 L12.end
  constraint coincident P1 L11.end
  constraint horizontal L34
  constraint vertical L35
  constraint horizontal L36
  constraint vertical L37
  constraint coincident L10 L35.end
  constraint coincident L9 L34.start
  constraint horizontal L38
  constraint vertical L39
  constraint horizontal L40
  constraint vertical L41
  constraint coincident L10 L39.end
  constraint coincident L31 L38.start
  measures "d219" distance of L30 L41
  measures "d220" distance of L32 L39
  measures "d221" distance of L8 L37
  measures "d222" distance of L0 L35
  measures "d223" distance of L3 L10
extrude "Extrude1'" add sketch "Sketch1 (2)" along normal blind 5 from surface at 0.5 separate body contours A0 L9 A9 L34 L35 L37 | A0 L10 A9 L35 L36 L37 | L10 L11 L12 L13 L26 L28 L29 L36 L40 | L10 L27 L33 L39 L40 L41 | L27 L31 L33 L38 L39 L41 | L14 L15 L16 L17 | L18 L19 L20 L21 | L22 L23 L24 L25 | A1 | A2 | A3 | A4 | A5 | A6 | A7 | A8 | A10 makes body 13 in component "Component"
extrude "Extrude2'" add 2 faces at (145.1667, -246.6728, 8.1667) (79.1667, -246.6728, 8.1667) along direction (0, -1, 0) blind 0.5 on bodies 13 bodies 13 in component "Component"
fillet "Fillet1" radius 3 2 edges at (146, -247.1728, 6.5) (80, -247.1728, 6.5) on bodies 13 in component "Component"
sketch "Sketch2 (2)" plane through (0, 0, 11.5) normal (0, 0, 1) x (-1, 0, 0) in component "Component"
  line L0 (-143.5, 226.6728) -> (-143.5, 247.1728)
  line L1 (-143.5, 247.1728) -> (-148.5, 247.1728)
  line L2 (-148.5, 247.1728) -> (-148.5, 226.6728)
  line L3 (-148.5, 226.6728) -> (-154, 226.6728)
  line L4 (-154, 226.6728) -> (-154, 188)
  line L5 (-154, 188) -> (-72, 188)
  line L6 (-72, 188) -> (-72, 226.6728)
  line L7 (-72, 226.6728) -> (-77.5, 226.6728)
  line L8 (-77.5, 226.6728) -> (-77.5, 247.1728)
  line L9 (-77.5, 247.1728) -> (-82.5, 247.1728)
  line L10 (-82.5, 247.1728) -> (-82.5, 226.6728)
  line L11 (-82.5, 226.6728) -> (-143.5, 226.6728)
  circle A0 centre (-80, 226.6728) radius 5
  line L12 (-77.5, 226.6728) -> (-80, 226.6728) construction
  line L13 (-80, 226.6728) -> (-82.5, 226.6728) construction
  circle A1 centre (-146, 226.6728) radius 5
  line L14 (-143.5, 226.6728) -> (-146, 226.6728) construction
  line L15 (-146, 226.6728) -> (-148.5, 226.6728) construction
  dimension "d230" = 10
  dimension "d231" = 10
  constraint coincident L7.end L8.start
  constraint coincident A0.centre L12.end
  constraint perpendicular L8 L12
  constraint coincident L10.end L11.start
  constraint equal L12 L13
  constraint coincident L0.start L11.end
  constraint coincident A1.centre L14.end
  constraint coincident L2.end L3.start
  constraint horizontal L15
  constraint equal L14 L15
  measures "d230" diameter of A0
  measures "d231" diameter of A1
extrude "Extrude3" cut sketch "Sketch2 (2)" along normal blind 2 from surface at -5 contours L3 L4 L5 L6 L7 L11 A0 A1 bodies 13 in component "Component"
sketch "Sketch3 (2)" plane through (154, 0, 0) normal (1, 0, 0) x (0, 1, 0) in component "Component"
  line L0 (-226.6728, 8.5) -> (-188, 8.5)
  line L1 (-188, 8.5) -> (-188, 11.5)
  line L2 (-188, 11.5) -> (-226.6728, 11.5)
  line L3 (-226.6728, 11.5) -> (-226.6728, 8.5)
  line L4 (-226.6728, 6.5) -> (-221.6728, 6.5)
  line L5 (-226.6728, 6.5) -> (-226.6728, 8.5)
  line L6 (-226.6728, 8.5) -> (-221.6728, 8.5)
  line L7 (-226.6728, 8.5) -> (-226.6728, 6.5)
  line L8 (-221.6728, 8.5) -> (-231.7618, 6.5)
  line L9 (-231.7618, 6.5) -> (-221.6728, 6.5)
  line L10 (-221.6728, 8.5) -> (-221.6728, 6.5)
  line L11 (-226.6728, 6.5) -> (-244.1728, 6.5)
  constraint coincident L6.end L8.start
  constraint coincident L4.end L9.end
  constraint coincident L8.end L11
extrude "Extrude4'" cut sketch "Sketch3 (2)" against normal blind 88 contours L4 L5 L7 L8 L9 L10 | L5 L7 L8 L9 L11 bodies 13 in component "Component"
sketch "Sketch4 (2)" plane through (0, 0, 8.5) normal (0, 0, -1) x (1, 0, 0) in component "Component"
  arc A0 (141, 226.6728) -> (146, 221.6728) centre (146, 226.6728) ccw
  line L0 (141, 226.6728) -> (85, 226.6728)
  arc A1 (80, 221.6728) -> (85, 226.6728) centre (80, 226.6728) ccw
  arc A2 (75, 226.6728) -> (80, 221.6728) centre (80, 226.6728) ccw
  line L1 (75, 226.6728) -> (72, 226.6728)
  line L2 (72, 226.6728) -> (72, 188)
  line L3 (72, 188) -> (154, 188)
  line L4 (154, 188) -> (154, 226.6728)
  line L5 (154, 226.6728) -> (151, 226.6728)
  arc A3 (146, 221.6728) -> (151, 226.6728) centre (146, 226.6728) ccw
  line L6 (72, 246.6728) -> (72, 188)
  line L7 (72, 188) -> (154, 188)
  line L8 (154, 188) -> (154, 246.6728)
  line L9 (154, 246.6728) -> (72, 246.6728)
  line L10 (133.7271, 200) -> (133.7271, 206)
  line L11 (133.7271, 206) -> (129.7271, 206)
  line L12 (129.7271, 206) -> (129.7271, 200)
  line L13 (129.7271, 200) -> (133.7271, 200)
  line L14 (108.7271, 200) -> (108.7271, 206)
  line L15 (108.7271, 206) -> (104.7271, 206)
  line L16 (104.7271, 206) -> (104.7271, 200)
  line L17 (104.7271, 200) -> (108.7271, 200)
  line L18 (83.7271, 200) -> (83.7271, 206)
  line L19 (83.7271, 206) -> (79.7271, 206)
  line L20 (79.7271, 206) -> (79.7271, 200)
  line L21 (79.7271, 200) -> (83.7271, 200)
  circle A4 centre (142.2021, 202.9356) radius 3.8
  circle A5 centre (106.2021, 209.4287) radius 2.8
  circle A6 centre (81.2021, 196.4356) radius 2.8
  circle A7 centre (106.2021, 196.4356) radius 2.8
  circle A8 centre (131.2021, 209.4287) radius 2.8
  circle A9 centre (117.2021, 202.9356) radius 3.8
  circle A10 centre (81.2021, 209.4287) radius 2.8
  circle A11 centre (92.2021, 202.9356) radius 3.8
  line L22 (72, 188) -> (72, 236.7154)
  arc A12 (100.5171, 241.6728) -> (72, 236.7154) centre (100.5171, 157.1728) ccw
  line L23 (100.5171, 241.6728) -> (154, 241.6728)
  line L24 (154, 241.6728) -> (154, 188)
  line L25 (154, 188) -> (72, 188)
  circle A13 centre (131.2021, 196.4356) radius 2.8
  line L26 (77.7271, 206) -> (75.7271, 206)
  line L27 (75.7271, 206) -> (75.7271, 200)
  line L28 (75.7271, 200) -> (77.7271, 200)
  line L29 (77.7271, 200) -> (77.7271, 206)
  line L30 (88.2021, 209.9356) -> (99.2021, 209.9356)
  line L31 (99.2021, 209.9356) -> (99.2021, 212.9356)
  line L32 (99.2021, 212.9356) -> (88.2021, 212.9356)
  line L33 (88.2021, 212.9356) -> (88.2021, 209.9356)
  line L34 (92.2021, 202.9356) -> (117.2021, 202.9356) construction
  line L35 (113.7021, 212.9356) -> (113.7021, 209.9356)
  line L36 (124.7021, 212.9356) -> (113.7021, 212.9356)
  line L37 (113.7021, 209.9356) -> (124.7021, 209.9356)
  line L38 (124.7021, 209.9356) -> (124.7021, 212.9356)
  line L39 (139.2021, 212.9356) -> (139.2021, 209.9356)
  line L40 (150.2021, 212.9356) -> (139.2021, 212.9356)
  line L41 (139.2021, 209.9356) -> (150.2021, 209.9356)
  line L42 (150.2021, 209.9356) -> (150.2021, 212.9356)
  line L43 (88.2021, 195.9356) -> (88.2021, 192.9356)
  line L44 (99.2021, 195.9356) -> (88.2021, 195.9356)
  line L45 (88.2021, 192.9356) -> (99.2021, 192.9356)
  line L46 (99.2021, 192.9356) -> (99.2021, 195.9356)
  line L47 (113.7021, 195.9356) -> (113.7021, 192.9356)
  line L48 (124.7021, 195.9356) -> (113.7021, 195.9356)
  line L49 (113.7021, 192.9356) -> (124.7021, 192.9356)
  line L50 (124.7021, 192.9356) -> (124.7021, 195.9356)
  line L51 (139.2021, 195.9356) -> (139.2021, 192.9356)
  line L52 (150.2021, 195.9356) -> (139.2021, 195.9356)
  line L53 (139.2021, 192.9356) -> (150.2021, 192.9356)
  line L54 (150.2021, 192.9356) -> (150.2021, 195.9356)
  line L55 (102.7271, 200) -> (102.7271, 206)
  line L56 (100.7271, 200) -> (102.7271, 200)
  line L57 (100.7271, 206) -> (100.7271, 200)
  line L58 (102.7271, 206) -> (100.7271, 206)
  line L59 (127.7271, 200) -> (127.7271, 206)
  line L60 (125.7271, 200) -> (127.7271, 200)
  line L61 (125.7271, 206) -> (125.7271, 200)
  line L62 (127.7271, 206) -> (125.7271, 206)
  dimension "d237" = 7
  dimension "d238" = 7
  dimension "d239" = 7
  dimension "d240" = 3
  dimension "d243" = 51
  dimension "d244" = -17
  dimension "d245" = 2
  dimension "d246" = 2
  dimension "d247" = 6
  dimension "d250" = 50
  dimension "d251" = 0
  constraint horizontal L26
  constraint vertical L27
  constraint horizontal L28
  constraint vertical L29
  constraint horizontal L30
  constraint vertical L31
  constraint horizontal L32
  constraint vertical L33
  constraint coincident A11.centre L34.start
  constraint coincident A9.centre L34.end
  constraint collinear L19 L26
  measures "d237" distance of A10.centre L33
  measures "d238" distance of A5.centre L31
  measures "d239" distance of L30 A11.centre
  measures "d240" distance of L30.end L31.end
  measures "d245" distance of L20 L29
  measures "d246" distance of L26.start L26.end
  measures "d247" distance of L26.end L27.end
extrude "Extrude5" add sketch "Sketch4 (2)" along normal up to surface (8.3 mm away) contours L26 L27 L28 L29 | L30 L31 L32 L33 | L35 L36 L37 L38 | L39 L40 L41 L42 | L43 L44 L45 L46 | L47 L48 L49 L50 | L51 L52 L53 L54 | L55 L56 L57 L58 | L59 L60 L61 L62 bodies 13 in component "Component"
sketch "Sketch5" plane through (77.5, 0, 0) normal (-1, 0, 0) x (0, -1, 0) in component "Component"
  line L0 (226.6728, 7.5088) -> (231.7618, 6.5)
  line L1 (231.7618, 6.5) -> (244.1728, 6.5)
  arc A0 (244.1728, 6.5) -> (247.1728, 9.5) centre (244.1728, 9.5) ccw
  line L2 (247.1728, 9.5) -> (247.1728, 11.5)
  line L3 (247.1728, 11.5) -> (226.6728, 11.5)
  line L4 (226.6728, 11.5) -> (226.6728, 7.5088)
  circle A1 centre (244.1728, 9) radius 1.7
extrude "Extrude7" cut sketch "Sketch5" against normal blind 112 contours A1 bodies 13 in component "Component"
sketch "Sketch13" plane through (0, 0, -2) normal (0, 0, -1) x (1, 0, 0)
  line L0 (72, 246.6728) -> (72, 188)
  line L1 (72, 188) -> (154, 188)
  line L2 (154, 188) -> (154, 246.6728)
  line L3 (154, 246.6728) -> (72, 246.6728)
  line L4 (72, 246.6728) -> (80.517, 246.6728)
  line L5 (80.517, 246.6728) -> (80.517, 254.0578)
  line L6 (80.517, 254.0578) -> (72, 254.0578)
  line L7 (72, 254.0578) -> (72, 246.6728)
  circle A0 centre (76.517, 250.0578) radius 1.6
  line L8 (144, 254.0578) -> (144, 246.6728)
  line L9 (152.517, 254.0578) -> (144, 254.0578)
  circle A1 centre (148.517, 250.0578) radius 1.6
  line L10 (152.517, 246.6728) -> (152.517, 254.0578)
  line L11 (144, 246.6728) -> (152.517, 246.6728)
  dimension "d283" = 3.2
  dimension "d284" = 3.385
  dimension "d287" = 4.517
  dimension "d288" = 4
  dimension "d289" = 4
  dimension "d292" = 72
  dimension "d293" = 0
  constraint horizontal L4
  constraint vertical L5
  constraint horizontal L6
  constraint vertical L7
  constraint coincident L0.start L3.end
  measures "d283" diameter of A0
  measures "d284" distance of L4 A0.centre
  measures "d287" distance of L7 A0.centre
  measures "d288" distance of L5 A0.centre
  measures "d289" distance of L6 A0.centre
extrude "Extrude17" add sketch "Sketch13" against normal blind 2.5 contours L3 L4 L5 L6 L7 | L3 L8 L9 L10 L11 bodies 1
fillet "Fillet2" radius 4 4 edges at (144, -254.0578, -0.75) (152.517, -254.0578, -0.75) (72, -254.0578, -0.75) (80.517, -254.0578, -0.75) on bodies 1
fillet "Fillet2" radius 4.5 1 edges at (80.517, -246.6728, -0.75) on bodies 1
fillet "Fillet2" radius 4.5 1 edges at (144, -246.6728, -0.75) on bodies 1
fillet "Fillet2" radius 4.75 1 edges at (152.517, -246.6728, -0.75) on bodies 1
fillet "Fillet2" radius 0.75 3 edges at (154, -246.6728, 3.55) (154, -244.1728, 11.6) (154, -241.6728, 4.55) on bodies 1
sketch "Sketch14" plane through (0, -188, 0) normal (0, 1, 0) x (-1, 0, 0)
  line L0 (-154, 8.5) -> (-72, 8.5)
  line L1 (-72, 8.5) -> (-72, 11.5)
  line L2 (-72, 11.5) -> (-154, 11.5)
  line L3 (-154, 11.5) -> (-154, 8.5)
  line L4 (-113, 24) -> (-113, -1) construction
  line L5 (-118, 11.5) -> (-108, 11.5)
  line L6 (-108, 11.5) -> (-108, 8.5)
  line L7 (-108, 8.5) -> (-118, 8.5)
  line L8 (-118, 8.5) -> (-118, 11.5)
  dimension "d299" = 5
  dimension "d300" = 5
  constraint vertical L4
  constraint midpoint L2 L4
  constraint horizontal L5
  constraint vertical L6
  constraint horizontal L7
  constraint vertical L8
  constraint coincident L0 L6.end
  constraint coincident L2 L5.start
  measures "d299" distance of L4 L6
  measures "d300" distance of L4 L8
extrude "Extrude8" add sketch "Sketch14" along normal blind 10 contours L0 L2 L5 L6 L7 L8 bodies 13 in component "Component"